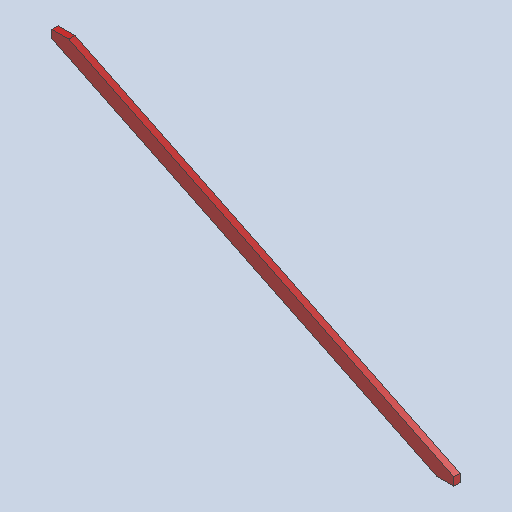
# Autodesk Inventor part: side1
Saved by Autodesk Inventor 2025.1 (Build 291241020, 241B)
## iProperties
Created: 2024-09-17
Part Number: side1
Material: Generic
Document SubType Name: Modeling
Designer: User
Density: 1 g/cm^3
Appearance: Default
Stock Number: 10
Author: User
Autodesk Inventor part; units mm, degrees
ref_plane "YZ Plane" through (0, 0, 0) normal (1, 0, 0) x (0, 1, 0)
ref_plane "XZ Plane" through (0, 0, 0) normal (0, 1, 0) x (-1, 0, 0)
ref_plane "XY Plane" through (0, 0, 0) normal (0, 0, 1) x (1, 0, 0)
sketch "Sketch1" plane through (0, 0, 0) normal (0, 0, 1) x (1, 0, 0)
  line L0 (0, -38.1) -> (2438.4, -38.1) projected
  line L1 (0, 2400.3) -> (0, -2476.5) projected
  line L2 (0, -1219.2) -> (2438.4, -1219.2) projected
  line L3 (2438.4, -1257.3) -> (2438.4, 2400.3) projected
  line L4 (2438.4, -1169.8101) -> (101.9663, -38.1)
  line L5 (0, -87.4899) -> (2336.4337, -1219.2)
  line L6 (101.9663, -38.1) -> (0, -38.1)
  line L7 (0, -87.4899) -> (0, -38.1)
  line L8 (2438.4, -1169.8101) -> (2438.4, -1219.2)
  line L9 (2336.4337, -1219.2) -> (2438.4, -1219.2)
  point P0 (0, 0)
  constraints: 12 end point, 4 collinear, 4 point on line, 1 parallel, 2 other
extrude "Extrusion1" add sketch "Sketch1" against normal blind 38.1 contours L0 L4 L3 L2 L5 L1
body "Solid1"
